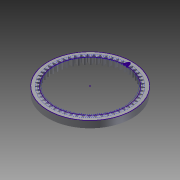
# Autodesk Inventor part: Z53
Saved by Autodesk Inventor 2014 (Build 180170000, 170)
## iProperties
Created: 2013-05-24
Part Number: Z53
Material: Generic
Document SubType Name: Modeling
Designer: hartmann
Density: 1 g/cm^3
Appearance: Default
Author: hartmann
Autodesk Inventor part; units mm, degrees
ref_plane "YZ Plane" through (0, 0, 0) normal (1, 0, 0) x (0, 1, 0)
ref_plane "XZ Plane" through (0, 0, 0) normal (0, 1, 0) x (-1, 0, 0)
ref_plane "XY Plane" through (0, 0, 0) normal (0, 0, 1) x (1, 0, 0)
sketch "Sketch1" plane through (0, 0, 0) normal (0, 0, 1) x (1, 0, 0)
  spline S0 degree 3 poles (-0.4266, 10.2394) (-0.4182, 10.2788) (-0.4014, 10.3576) (-0.3697, 10.4742) (-0.3341, 10.5897) (-0.2946, 10.7039) (-0.2516, 10.8168) (-0.1903, 10.9659) (-0.1384, 11.075) (-0.1037, 11.1478) knots 0 0 0 0 0.012083 0.024166 0.036249 0.048332 0.060415 0.072499 0.096663 0.096663 0.096663 0.096663
  spline S1 degree 3 poles (0.4266, 10.2394) (0.4182, 10.2788) (0.4014, 10.3576) (0.3697, 10.4742) (0.3341, 10.5897) (0.2946, 10.7039) (0.2516, 10.8168) (0.1903, 10.9659) (0.1384, 11.075) (0.1037, 11.1478) knots 0 0 0 0 0.012083 0.024166 0.036249 0.048332 0.060415 0.072499 0.096663 0.096663 0.096663 0.096663
  circle A0 centre (0, 0) radius 11.1482 construction
  circle A1 centre (0, 0) radius 9.9607 construction
  circle A2 centre (0, 0) radius 10.6 construction
  circle A3 centre (0, 0) radius 10.2482
  circle A4 centre (0, 0) radius 12.0482
  arc A5 (0.1037, 11.1478) -> (-0.1037, 11.1478) centre (0, 0) ccw
  point P0 (-0.4003, 10.3573)
  point P1 (-0.3691, 10.474)
  point P2 (-0.3335, 10.5895)
  point P3 (-0.294, 10.7037)
  point P4 (-0.2511, 10.8167)
  point P5 (-0.205, 10.9283)
  point P6 (0.4003, 10.3573)
  point P7 (0.3691, 10.474)
  point P8 (0.3335, 10.5895)
  point P9 (0.294, 10.7037)
  point P10 (0.2511, 10.8167)
  point P11 (0.205, 10.9283)
  constraints: 6 centre point, 6 point on circle, 39 other
extrude "Extrusion1" add sketch "Sketch1" against normal blind 2 contours S0 A5 S1 A3 | A4
extrude "Extrusion2" cut sketch "Sketch1" against normal through all contours S0 A5 S1 A3
pattern_circular "Runde Anordnung1" count 53 over 360 about axis through (0, 0, -10) along (0, 0, 1) of "Extrusion2"
equation "\"d0\" = Zahnbreite"
equation "\"Modul\" = 0.4"
equation "\"Druckwinkel\" = 20deg"
equation "\"UnitProfileClearance\" = 0.25"
equation "\"UnitRoundRadius\" = 0.35"
equation "\"Kopfdurchmesser\" = 20.49648"
equation "\"Stammdurchmesser\" = 22.29648"
equation "\"Grundkreisdurchmesser\" = 19.92148"
equation "\"Gewindedurchmesser\" = 21.2"
equation "\"Zahnbreite\" = 2"
equation "\"Schrägungswinkel\" = 0"
equation "\"UnitCorrection\" = 0.1206"
equation "\"UnitAddendumModification\" = 0"
equation "\"Zahnkreisteilung\" = 1.25664"
equation "\"UnitBacklashShift\" = 0"
equation "\"Gesamtzahnstärke\" = 0.04824"
